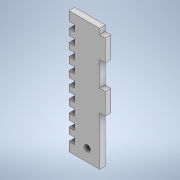
# Autodesk Inventor part: rail
Saved by Autodesk Inventor 2020 (Build 240168000, 168)
## iProperties
Created: 2019-12-19
Part Number: rail
Material: Générique
Document SubType Name: Modeling
Designer: damien
Density: 1 g/cm^3
Appearance: Par défaut
Author: damien
Autodesk Inventor part; units mm, degrees
ref_plane "YZ Plane" through (0, 0, 0) normal (1, 0, 0) x (0, 1, 0)
ref_plane "XZ Plane" through (0, 0, 0) normal (0, 1, 0) x (-1, 0, 0)
ref_plane "XY Plane" through (0, 0, 0) normal (0, 0, 1) x (1, 0, 0)
sketch "Esquisse1" plane through (0, 0, 0) normal (0, 0, 1) x (1, 0, 0)
  line L0 (0, 240) -> (-100, 240)
  line L1 (-100, 240) -> (-100, -160)
  line L2 (-100, -160) -> (0, -160)
  line L3 (0, -160) -> (0, 0)
  line L4 (0, 0) -> (18.55, 0)
  line L5 (18.55, 0) -> (18.55, 70)
  line L6 (18.55, 70) -> (0, 70)
  line L7 (0, 70) -> (0, 151.45)
  line L8 (0, 151.45) -> (18.55, 151.45)
  line L9 (18.55, 151.45) -> (18.55, 221.45)
  line L10 (18.55, 221.45) -> (0, 221.45)
  line L11 (0, 221.45) -> (0, 240)
  dimension "d0" = 400
  dimension "d1" = 70
  dimension "d2" = 70
  dimension "d3" = 100
  dimension "d4" = 160
  dimension "d5" = 81.45
  dimension "d6" = 18.55
  constraints: 24 end point, 9 perpendicular, 3 point on line, 1 collinear, 1 horizontal, 1 vertical
  measures "d0" distance of L0.end L1.end
  measures "d1" distance of L4.end L5.end
  measures "d2" distance between parallel lines of L8 L10
  measures "d3" distance of L0.start L0.end
  measures "d4" distance of L2.end L3.end
  measures "d5" distance between parallel lines of L6 L8
  measures "d6" distance between parallel lines of L7 L5
extrude "Extrusion1" add sketch "Esquisse1" along normal blind 18.55
sketch "Esquisse2" plane through (0, 0, 18.55) normal (0, 0, 1) x (1, 0, 0)
  line L0 (-100, 210) -> (-81.45, 210)
  line L1 (-81.45, 210) -> (-81.45, 190)
  line L2 (-81.45, 190) -> (-100, 190)
  line L3 (-100, 190) -> (-100, 210)
  line L4 (0, 240) -> (-100, 240) projected
  line L5 (-100, 240) -> (-100, -160) projected
  line L6 (-100, 170) -> (-81.45, 170)
  line L7 (-81.45, 170) -> (-81.45, 150)
  line L8 (-81.45, 150) -> (-100, 150)
  line L9 (-100, 150) -> (-100, 170)
  line L10 (-100, 130) -> (-81.45, 130)
  line L11 (-81.45, 130) -> (-81.45, 110)
  line L12 (-81.45, 110) -> (-100, 110)
  line L13 (-100, 110) -> (-100, 130)
  line L14 (-100, 90) -> (-81.45, 90)
  line L15 (-81.45, 90) -> (-81.45, 70)
  line L16 (-81.45, 70) -> (-100, 70)
  line L17 (-100, 70) -> (-100, 90)
  line L18 (-100, 50) -> (-81.45, 50)
  line L19 (-81.45, 50) -> (-81.45, 30)
  line L20 (-81.45, 30) -> (-100, 30)
  line L21 (-100, 30) -> (-100, 50)
  line L22 (-100, 10) -> (-81.45, 10)
  line L23 (-81.45, 10) -> (-81.45, -10)
  line L24 (-81.45, -10) -> (-100, -10)
  line L25 (-100, -10) -> (-100, 10)
  line L26 (-100, -30) -> (-81.45, -30)
  line L27 (-81.45, -30) -> (-81.45, -50)
  line L28 (-81.45, -50) -> (-100, -50)
  line L29 (-100, -50) -> (-100, -30)
  line L30 (-100, -70) -> (-81.45, -70)
  line L31 (-81.45, -70) -> (-81.45, -90)
  line L32 (-81.45, -90) -> (-100, -90)
  line L33 (-100, -90) -> (-100, -70)
  line L34 (-100, -110) -> (-81.45, -110)
  line L35 (-81.45, -110) -> (-81.45, -130)
  line L36 (-81.45, -130) -> (-100, -130)
  line L37 (-100, -130) -> (-100, -110)
  point P0 (0, 0)
  dimension "d9" = 30
  dimension "d10" = 20
  dimension "d11" = 18.55
  dimension "d14" = 40
  constraints: 72 end point, 2 parallel, 1 collinear, 1 horizontal, 1 perpendicular, 1 vertical, 64 other
  measures "d9" distance between parallel lines of L4 L0
  measures "d10" distance of L2.end L0.start
  measures "d11" distance of L1.end L2.end
  measures "d14" distance of L0.start L6.start
extrude "Extrusion2" cut sketch "Esquisse2" against normal blind 18.55
sketch "Esquisse3" plane through (0, 0, 18.55) normal (0, 0, 1) x (1, 0, 0)
  circle A0 centre (-40, -120) radius 10
  line L0 (0, -160) -> (0, 0) projected
  line L1 (-100, -160) -> (0, -160) projected
  dimension "d21" = 40
  dimension "d22" = 20
  dimension "d23" = 40
  constraints: 1 centre point
  measures "d21" distance from line of L0 A0.centre
  measures "d22" diameter of A0
  measures "d23" distance from line of L1 A0.centre
extrude "Extrusion3" cut sketch "Esquisse3" against normal blind 18.55
